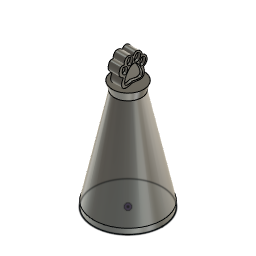
Pawn v1 (Autodesk Fusion 360 design; units mm, degrees)
Autodesk Fusion 360 part; units mm, degrees
sketch "Sketch1" plane through (0, 0, 0) normal (0, 0, 1) x (1, 0, 0)
  circle A0 centre (0, 0) radius 12.5
  dimension "d1" = 25
  constraint coincident A0.centre origin
  measures "d1" diameter of A0
extrude "Extrude2" add sketch "Sketch1" along normal blind 2 makes body 1
ref_plane "WorkPlane3" through (0, 0, 22) normal (0, 0, 1) x (1, 0, 0)
sketch "Sketch5" plane through (0, 0, 22) normal (0, 0, 1) x (1, 0, 0)
ref_plane "WorkPlane4" through (0, 0, 37) normal (0, 0, 1) x (1, 0, 0)
sketch "Sketch6" plane through (0, 0, 37) normal (0, 0, 1) x (1, 0, 0)
  circle A0 centre (0, 0) radius 5
  dimension "d11" = 10
  constraint coincident A0.centre origin
  measures "d11" diameter of A0
loft "Loft2" add profiles "Sketch6" section 1 section 2 face at (-3.3879, -0.621, 2) on bodies 1 bodies 1
sphere "SpherePrimitive1" add diameter 16 placed x (1, 0, 0) y (0, 0, -1) z (0, 1, 0) at (-0.1087, 0, 43.069) separate body makes body 2
move_body "Move1" bodies 2 to x (1, 0, 0) y (0, 1, 0) z (0, 0, 1) at (0, 0, 2)
ref_plane "WorkPlane5" through (0, 0, 40) normal (0, 0, 1) x (1, 0, 0)
ref_plane "WorkPlane6" through (0, 0, 40) normal (0, 0, 1) x (1, 0, 0)
sketch "Sketch9" plane through (0, 0, 40) normal (0, 0, 1) x (1, 0, 0)
  circle A0 centre (0, 0) radius 5.75
  dimension "d15" = 11.5
  constraint coincident A0.centre origin
  measures "d15" diameter of A0
loft "Loft3" add profiles "Sketch9" section 1 section 2 face at (1.3101, -1.9935, 37) on bodies 1 bodies 1
sketch "Sketch10" plane through (0, 0, 0) normal (1, 0, 0) x (0, 1, 0)
sketch "Sketch11" plane through (0, 0, 0) normal (1, 0, 0) x (0, 1, 0)
  spline S0 degree 5 poles (-3.2787, 40.0454) (-3.329, 40.0614) (-3.4264, 40.0962) (-3.5629, 40.1571) (-3.7251, 40.2561) (-3.8983, 40.4129) (-4.046, 40.6065) (-4.1701, 40.8394) (-4.2671, 41.1119) (-4.3286, 41.421) (-4.346, 41.7602) (-4.3129, 42.1194) (-4.2293, 42.4841) (-4.1045, 42.8352) (-3.9605, 43.1487) (-3.8264, 43.402) (-3.7324, 43.5808) (-3.7041, 43.6847) (-3.7567, 43.7354) (-3.8898, 43.7779) (-4.0914, 43.8587) (-4.3385, 44.0022) (-4.6016, 44.2078) (-4.8494, 44.461) (-5.0537, 44.7411) (-5.1943, 45.0301) (-5.2638, 45.3212) (-5.2715, 45.6253) (-5.2323, 45.9576) (-5.1613, 46.3292) (-5.0588, 46.7299) (-4.9167, 47.132) (-4.6743, 47.4432) (-4.3169, 47.6052) (-3.9101, 47.6407) (-3.5409, 47.6019) (-3.2925, 47.5555) (-3.2103, 47.5569) (-3.2577, 47.6187) (-3.3419, 47.7258) (-3.4015, 47.8936) (-3.4041, 48.1515) (-3.3297, 48.5128) (-3.1643, 48.9586) (-2.8776, 49.3926) (-2.4359, 49.6631) (-1.8831, 49.7359) (-1.2904, 49.6236) (-0.7461, 49.3872) (-0.3293, 49.108) (-0.0883, 48.8721) (-0.0225, 48.7508) (-0.0481, 48.7788) (-0.0376, 48.9475) (0.0779, 49.2091) (0.3231, 49.4918) (0.6879, 49.7166) (1.1382, 49.8139) (1.6263, 49.7381) (2.102, 49.4885) (2.5203, 49.1092) (2.8455, 48.6689) (3.056, 48.2458) (3.1485, 47.9102) (3.1443, 47.7074) (3.0901, 47.6442) (3.0717, 47.6629) (3.173, 47.6744) (3.413, 47.6175) (3.7661, 47.4522) (4.1752, 47.1612) (4.568, 46.7471) (4.8713, 46.2325) (5.0266, 45.6568) (5.0053, 45.0802) (4.8255, 44.5564) (4.5349, 44.1273) (4.1987, 43.8196) (3.8857, 43.6405) (3.6544, 43.573) (3.5411, 43.5739) (3.5419, 43.5636) (3.6213, 43.453) (3.7415, 43.2023) (3.8648, 42.8146) (3.9562, 42.323) (3.9849, 41.78) (3.9268, 41.2459) (3.7666, 40.778) (3.4996, 40.4189) (3.1339, 40.1852) (2.6877, 40.0725) (2.1856, 40.0606) (1.6557, 40.1193) (1.1259, 40.2132) (0.6213, 40.3077) (0.1604, 40.3737) (-0.248, 40.3937) (-0.607, 40.3654) (-0.9274, 40.2973) (-1.2242, 40.2048) (-1.5129, 40.1065) (-1.806, 40.0204) (-2.1092, 39.96) (-2.4188, 39.9314) (-2.7258, 39.936) (-2.9602, 39.9652) (-3.1247, 40.0003) (-3.2284, 40.0294) (-3.2787, 40.0454) knots 0 0 0 0 0 0 0.00952381 0.01904762 0.02857143 0.03809524 0.04761905 0.05714286 0.06666667 0.07619048 0.08571429 0.0952381 0.1047619 0.11428571 0.12380952 0.13333333 0.14285714 0.15238095 0.16190476 0.17142857 0.18095238 0.19047619 0.2 0.20952381 0.21904762 0.22857143 0.23809524 0.24761905 0.25714286 0.26666667 0.27619048 0.28571429 0.2952381 0.3047619 0.31428571 0.32380952 0.33333333 0.34285714 0.35238095 0.36190476 0.37142857 0.38095238 0.39047619 0.4 0.40952381 0.41904762 0.42857143 0.43809524 0.44761905 0.45714286 0.46666667 0.47619048 0.48571429 0.4952381 0.5047619 0.51428571 0.52380952 0.53333333 0.54285714 0.55238095 0.56190476 0.57142857 0.58095238 0.59047619 0.6 0.60952381 0.61904762 0.62857143 0.63809524 0.64761905 0.65714286 0.66666667 0.67619048 0.68571429 0.6952381 0.7047619 0.71428571 0.72380952 0.73333333 0.74285714 0.75238095 0.76190476 0.77142857 0.78095238 0.79047619 0.8 0.80952381 0.81904762 0.82857143 0.83809524 0.84761905 0.85714286 0.86666667 0.87619048 0.88571429 0.8952381 0.9047619 0.91428571 0.92380952 0.93333333 0.94285714 0.95238095 0.96190476 0.97142857 0.98095238 0.99047619 1 1 1 1 1 1
  line L0 (-4.3951, 46.9042) -> (-1.7589, 51.2055)
  line L1 (-6.0697, 44.8771) -> (-3.7447, 49.286)
  line L2 (4.2895, 48.7822) -> (5.6048, 42.9491)
  point P0 (-4.0893, 40.6991)
  point P1 (-4.2201, 42.4774)
  point P2 (-3.7232, 43.6541)
  point P3 (-3.9799, 43.8169)
  point P4 (-5.1582, 44.9824)
  point P5 (-4.9072, 47.0816)
  point P6 (-3.2787, 47.5628)
  point P7 (-3.2787, 47.6466)
  point P8 (-3.077, 49.0548)
  point P9 (-0.0768, 48.8344)
  point P10 (-0.0396, 48.8147)
  point P11 (1.3943, 49.7526)
  point P12 (3.1219, 47.7028)
  point P13 (3.0986, 47.6608)
  point P14 (4.9471, 45.8656)
  point P15 (3.6234, 43.5786)
  point P16 (3.5674, 43.5289)
  point P17 (3.7321, 40.79)
  point P18 (0.2661, 40.3525)
  point P19 (-1.7349, 40.0454)
  constraint midpoint P8 L0
  constraint midpoint P5 L1
  constraint midpoint P14 L2
extrude "Extrude3" add sketch "Sketch11" along normal mid plane 4 separate body contours S0 makes body 3
sketch "Sketch12" plane through (2, 0, 0) normal (1, 0, 0) x (0, 1, 0)
  spline S0 degree 5 poles (-3.2787, 40.0454) (-3.2284, 40.0294) (-3.1247, 40.0003) (-2.9602, 39.9652) (-2.7258, 39.936) (-2.4188, 39.9314) (-2.1092, 39.96) (-1.806, 40.0204) (-1.5129, 40.1065) (-1.2242, 40.2048) (-0.9274, 40.2973) (-0.607, 40.3654) (-0.248, 40.3937) (0.1604, 40.3737) (0.6213, 40.3077) (1.1259, 40.2132) (1.6557, 40.1193) (2.1856, 40.0606) (2.6877, 40.0725) (3.1339, 40.1852) (3.4996, 40.4189) (3.7666, 40.778) (3.9268, 41.2459) (3.9849, 41.78) (3.9562, 42.323) (3.8648, 42.8146) (3.7415, 43.2023) (3.6213, 43.453) (3.5419, 43.5636) (3.5411, 43.5739) (3.6544, 43.573) (3.8857, 43.6405) (4.1987, 43.8196) (4.5349, 44.1273) (4.8255, 44.5564) (5.0053, 45.0802) (5.0266, 45.6568) (4.8713, 46.2325) (4.568, 46.7471) (4.1752, 47.1612) (3.7661, 47.4522) (3.413, 47.6175) (3.207, 47.6664) (3.1242, 47.6667) (3.0991, 47.6613) (3.0931, 47.6593) (3.0922, 47.6589) knots -1 -1 -1 -1 -1 -1 -0.990476 -0.980952 -0.971429 -0.961905 -0.952381 -0.942857 -0.933333 -0.92381 -0.914286 -0.904762 -0.895238 -0.885714 -0.87619 -0.866667 -0.857143 -0.847619 -0.838095 -0.828571 -0.819048 -0.809524 -0.8 -0.790476 -0.780952 -0.771429 -0.761905 -0.752381 -0.742857 -0.733333 -0.72381 -0.714286 -0.704762 -0.695238 -0.685714 -0.67619 -0.666667 -0.657143 -0.647619 -0.638095 -0.628571 -0.619048 -0.609524 -0.606751 -0.606751 -0.606751 -0.606751 -0.606751 -0.606751
  spline S1 degree 5 poles (3.0922, 47.6589) (3.0916, 47.6586) (3.0911, 47.6584) (3.0908, 47.6582) (3.0906, 47.6582) (3.0906, 47.6582) knots 0.602912 0.602912 0.602912 0.602912 0.602912 0.602912 0.604832 0.604832 0.604832 0.604832 0.604832 0.604832
  spline S2 degree 5 poles (3.0922, 47.6589) (3.093, 47.6595) (3.098, 47.6627) (3.1148, 47.6778) (3.1449, 47.7356) (3.1485, 47.9102) (3.056, 48.2458) (2.8455, 48.6689) (2.5203, 49.1092) (2.102, 49.4885) (1.6263, 49.7381) (1.1382, 49.8139) (0.6879, 49.7166) (0.3231, 49.4918) (0.0779, 49.2091) (-0.0376, 48.9475) (-0.0481, 48.7788) (-0.0225, 48.7508) (-0.0883, 48.8721) (-0.3293, 49.108) (-0.7461, 49.3872) (-1.2904, 49.6236) (-1.8831, 49.7359) (-2.4359, 49.6631) (-2.8776, 49.3926) (-3.1643, 48.9586) (-3.3297, 48.5128) (-3.4041, 48.1515) (-3.4015, 47.8936) (-3.3419, 47.7258) (-3.2577, 47.6187) (-3.2103, 47.5569) (-3.2925, 47.5555) (-3.5409, 47.6019) (-3.9101, 47.6407) (-4.3169, 47.6052) (-4.6743, 47.4432) (-4.9167, 47.132) (-5.0588, 46.7299) (-5.1613, 46.3292) (-5.2323, 45.9576) (-5.2715, 45.6253) (-5.2638, 45.3212) (-5.1943, 45.0301) (-5.0537, 44.7411) (-4.8494, 44.461) (-4.6016, 44.2078) (-4.3385, 44.0022) (-4.0914, 43.8587) (-3.8898, 43.7779) (-3.7567, 43.7354) (-3.7041, 43.6847) (-3.7324, 43.5808) (-3.8264, 43.402) (-3.9605, 43.1487) (-4.1045, 42.8352) (-4.2293, 42.4841) (-4.3129, 42.1194) (-4.346, 41.7602) (-4.3286, 41.421) (-4.2671, 41.1119) (-4.1701, 40.8394) (-4.046, 40.6065) (-3.8983, 40.4129) (-3.7251, 40.2561) (-3.5629, 40.1571) (-3.4264, 40.0962) (-3.329, 40.0614) (-3.2787, 40.0454) knots -0.6029125 -0.6029125 -0.6029125 -0.6029125 -0.6029125 -0.6029125 -0.6 -0.59047619 -0.58095238 -0.57142857 -0.56190476 -0.55238095 -0.54285714 -0.53333333 -0.52380952 -0.51428571 -0.5047619 -0.4952381 -0.48571429 -0.47619048 -0.46666667 -0.45714286 -0.44761905 -0.43809524 -0.42857143 -0.41904762 -0.40952381 -0.4 -0.39047619 -0.38095238 -0.37142857 -0.36190476 -0.35238095 -0.34285714 -0.33333333 -0.32380952 -0.31428571 -0.3047619 -0.2952381 -0.28571429 -0.27619048 -0.26666667 -0.25714286 -0.24761905 -0.23809524 -0.22857143 -0.21904762 -0.20952381 -0.2 -0.19047619 -0.18095238 -0.17142857 -0.16190476 -0.15238095 -0.14285714 -0.13333333 -0.12380952 -0.11428571 -0.1047619 -0.0952381 -0.08571429 -0.07619048 -0.06666667 -0.05714286 -0.04761905 -0.03809524 -0.02857143 -0.01904762 -0.00952381 0 0 0 0 0 0
  spline S3 degree 5 poles (-3.2297, 41.5048) (-3.2452, 41.6006) (-3.2623, 41.8061) (-3.2457, 42.155) (-3.1382, 42.691) (-2.8727, 43.4345) (-2.4965, 44.1953) (-2.0362, 44.9126) (-1.5214, 45.5276) (-0.9815, 45.9909) (-0.4424, 46.2689) (0.077, 46.3523) (0.5652, 46.2543) (1.0161, 46.0028) (1.4279, 45.6334) (1.8016, 45.1835) (2.1396, 44.6841) (2.4446, 44.1565) (2.7175, 43.6152) (2.9562, 43.0715) (3.1541, 42.5358) (3.2984, 42.0212) (3.3682, 41.5458) (3.334, 41.1358) (3.1675, 40.818) (2.8534, 40.6125) (2.3983, 40.5259) (1.8441, 40.5432) (1.2558, 40.6325) (0.7041, 40.7544) (0.2482, 40.8694) (-0.0789, 40.9452) (-0.2918, 40.9665) (-0.4526, 40.9375) (-0.6349, 40.8731) (-0.8899, 40.7913) (-1.2271, 40.709) (-1.6295, 40.6444) (-2.0617, 40.6189) (-2.4809, 40.6591) (-2.8451, 40.797) (-3.0621, 41.0082) (-3.1695, 41.2314) (-3.2142, 41.409) (-3.2297, 41.5048) knots 0 0 0 0 0 0 0.025 0.05 0.075 0.1 0.125 0.15 0.175 0.2 0.225 0.25 0.275 0.3 0.325 0.35 0.375 0.4 0.425 0.45 0.475 0.5 0.525 0.55 0.575 0.6 0.625 0.65 0.675 0.7 0.725 0.75 0.775 0.8 0.825 0.85 0.875 0.9 0.925 0.95 0.975 1 1 1 1 1 1
  spline S4 degree 5 poles (-3.7437, 46.842) (-3.718, 46.8616) (-3.6659, 46.8927) (-3.5864, 46.9161) (-3.4795, 46.91) (-3.3455, 46.8724) (-3.2102, 46.8341) (-3.0717, 46.8093) (-2.9283, 46.787) (-2.7794, 46.7437) (-2.627, 46.6532) (-2.4764, 46.497) (-2.3377, 46.2748) (-2.2233, 45.9989) (-2.1461, 45.69) (-2.1179, 45.373) (-2.147, 45.0729) (-2.236, 44.8093) (-2.3814, 44.5951) (-2.5749, 44.4385) (-2.8042, 44.3439) (-3.0544, 44.3137) (-3.3091, 44.3499) (-3.551, 44.4549) (-3.764, 44.629) (-3.9342, 44.8691) (-4.0514, 45.1667) (-4.1104, 45.506) (-4.1132, 45.8617) (-4.067, 46.2029) (-3.9823, 46.4988) (-3.8935, 46.6788) (-3.8201, 46.7752) (-3.7694, 46.8225) (-3.7437, 46.842) knots 0 0 0 0 0 0 0.033333 0.066667 0.1 0.133333 0.166667 0.2 0.233333 0.266667 0.3 0.333333 0.366667 0.4 0.433333 0.466667 0.5 0.533333 0.566667 0.6 0.633333 0.666667 0.7 0.733333 0.766667 0.8 0.833333 0.866667 0.9 0.933333 0.966667 1 1 1 1 1 1
  spline S5 degree 5 poles (-1.6285, 48.9967) (-1.5819, 49.0042) (-1.484, 49.0136) (-1.3243, 49.0106) (-1.0928, 48.9719) (-0.7997, 48.8653) (-0.5341, 48.7022) (-0.3245, 48.4873) (-0.1913, 48.2283) (-0.139, 47.938) (-0.158, 47.6326) (-0.2306, 47.3298) (-0.3365, 47.047) (-0.4579, 46.7993) (-0.5853, 46.5976) (-0.7218, 46.4468) (-0.8763, 46.348) (-1.0578, 46.3002) (-1.2699, 46.3017) (-1.5037, 46.3525) (-1.7406, 46.453) (-1.9583, 46.6032) (-2.1359, 46.8011) (-2.2591, 47.0414) (-2.326, 47.3139) (-2.3434, 47.605) (-2.323, 47.8994) (-2.2764, 48.1814) (-2.2111, 48.4366) (-2.1255, 48.6536) (-2.0091, 48.8248) (-1.882, 48.9209) (-1.7638, 48.9686) (-1.6752, 48.9892) (-1.6285, 48.9967) knots 0 0 0 0 0 0 0.033333 0.066667 0.1 0.133333 0.166667 0.2 0.233333 0.266667 0.3 0.333333 0.366667 0.4 0.433333 0.466667 0.5 0.533333 0.566667 0.6 0.633333 0.666667 0.7 0.733333 0.766667 0.8 0.833333 0.866667 0.9 0.933333 0.966667 1 1 1 1 1 1
  spline S6 degree 5 poles (1.554, 48.9967) (1.5157, 49.0039) (1.4395, 49.0119) (1.3271, 49.004) (1.1816, 48.9521) (1.007, 48.8205) (0.84, 48.6289) (0.6831, 48.387) (0.5439, 48.1068) (0.4346, 47.8012) (0.3687, 47.4845) (0.359, 47.1715) (0.4147, 46.8775) (0.5386, 46.618) (0.7246, 46.4083) (0.959, 46.2623) (1.2242, 46.1906) (1.5005, 46.1986) (1.7693, 46.2849) (2.016, 46.4394) (2.2294, 46.6452) (2.4019, 46.8826) (2.5284, 47.1323) (2.6065, 47.3786) (2.6351, 47.6135) (2.6152, 47.8366) (2.5493, 48.051) (2.4418, 48.26) (2.299, 48.4635) (2.1294, 48.6543) (1.9424, 48.8193) (1.7864, 48.9188) (1.6695, 48.9686) (1.5924, 48.9895) (1.554, 48.9967) knots 0 0 0 0 0 0 0.033333 0.066667 0.1 0.133333 0.166667 0.2 0.233333 0.266667 0.3 0.333333 0.366667 0.4 0.433333 0.466667 0.5 0.533333 0.566667 0.6 0.633333 0.666667 0.7 0.733333 0.766667 0.8 0.833333 0.866667 0.9 0.933333 0.966667 1 1 1 1 1 1
  spline S7 degree 5 poles (3.4122, 46.842) (3.3551, 46.8469) (3.2415, 46.8457) (3.0754, 46.8119) (2.8703, 46.7064) (2.655, 46.4928) (2.4899, 46.2215) (2.3796, 45.9175) (2.3246, 45.6023) (2.3213, 45.2902) (2.3643, 44.991) (2.4472, 44.7125) (2.5644, 44.4624) (2.7127, 44.2509) (2.8922, 44.093) (3.1036, 44.0045) (3.3442, 43.9992) (3.6056, 44.0856) (3.8696, 44.2632) (4.1107, 44.5228) (4.3016, 44.8487) (4.4178, 45.2193) (4.4416, 45.6092) (4.368, 45.9898) (4.2064, 46.3314) (3.976, 46.606) (3.7566, 46.7536) (3.5843, 46.8168) (3.4693, 46.8372) (3.4122, 46.842) knots 0 0 0 0 0 0 0.04 0.08 0.12 0.16 0.2 0.24 0.28 0.32 0.36 0.4 0.44 0.48 0.52 0.56 0.6 0.64 0.68 0.72 0.76 0.8 0.84 0.88 0.92 0.96 1 1 1 1 1 1
  point P0 (-0.7785, 46.0711)
  point P1 (1.6924, 45.3002)
  point P2 (3.2738, 42.0583)
  point P3 (2.7401, 40.6153)
  point P4 (0.0517, 40.9118)
  point P5 (-0.5809, 40.892)
  point P6 (-1.9448, 40.6351)
  point P7 (-3.2297, 46.842)
  point P8 (-2.6367, 46.6444)
  point P9 (-2.1425, 45.2013)
  point P10 (-2.9925, 44.3316)
  point P11 (-4.0533, 45.2409)
  point P12 (-0.2843, 48.3839)
  point P13 (-0.4425, 46.842)
  point P14 (-1.1146, 46.3083)
  point P15 (-2.1425, 46.842)
  point P16 (-2.2413, 48.3048)
  point P17 (0.7633, 48.5025)
  point P18 (0.4471, 46.842)
  point P19 (1.554, 46.2293)
  point P20 (2.5622, 47.2572)
  point P21 (2.404, 48.3048)
  point P22 (2.404, 45.9525)
  point P23 (2.5622, 44.4897)
  point P24 (3.4122, 44.0351)
  point P25 (4.4203, 45.4781)
extrude "Extrude4" cut sketch "Sketch12" against normal blind 1 contours S3 | S4 | S5 | S6 | S7 bodies 3
sketch "Sketch13" plane through (-2, 0, 0) normal (-1, 0, 0) x (0, -1, 0)
  spline S0 degree 5 poles (-3.0922, 47.6589) (-3.0931, 47.6593) (-3.0991, 47.6613) (-3.1242, 47.6667) (-3.207, 47.6664) (-3.413, 47.6175) (-3.7661, 47.4522) (-4.1752, 47.1612) (-4.568, 46.7471) (-4.8713, 46.2325) (-5.0266, 45.6568) (-5.0053, 45.0802) (-4.8255, 44.5564) (-4.5349, 44.1273) (-4.1987, 43.8196) (-3.8857, 43.6405) (-3.6544, 43.573) (-3.5411, 43.5739) (-3.5419, 43.5636) (-3.6213, 43.453) (-3.7415, 43.2023) (-3.8648, 42.8146) (-3.9562, 42.323) (-3.9849, 41.78) (-3.9268, 41.2459) (-3.7666, 40.778) (-3.4996, 40.4189) (-3.1339, 40.1852) (-2.6877, 40.0725) (-2.1856, 40.0606) (-1.6557, 40.1193) (-1.1259, 40.2132) (-0.6213, 40.3077) (-0.1604, 40.3737) (0.248, 40.3937) (0.607, 40.3654) (0.9274, 40.2973) (1.2242, 40.2048) (1.5129, 40.1065) (1.806, 40.0204) (2.1092, 39.96) (2.4188, 39.9314) (2.7258, 39.936) (2.9602, 39.9652) (3.1247, 40.0003) (3.2284, 40.0294) (3.2787, 40.0454) knots 0.606751 0.606751 0.606751 0.606751 0.606751 0.606751 0.609524 0.619048 0.628571 0.638095 0.647619 0.657143 0.666667 0.67619 0.685714 0.695238 0.704762 0.714286 0.72381 0.733333 0.742857 0.752381 0.761905 0.771429 0.780952 0.790476 0.8 0.809524 0.819048 0.828571 0.838095 0.847619 0.857143 0.866667 0.87619 0.885714 0.895238 0.904762 0.914286 0.92381 0.933333 0.942857 0.952381 0.961905 0.971429 0.980952 0.990476 1 1 1 1 1 1
  spline S1 degree 5 poles (3.2787, 40.0454) (3.329, 40.0614) (3.4264, 40.0962) (3.5629, 40.1571) (3.7251, 40.2561) (3.8983, 40.4129) (4.046, 40.6065) (4.1701, 40.8394) (4.2671, 41.1119) (4.3286, 41.421) (4.346, 41.7602) (4.3129, 42.1194) (4.2293, 42.4841) (4.1045, 42.8352) (3.9605, 43.1487) (3.8264, 43.402) (3.7324, 43.5808) (3.7041, 43.6847) (3.7567, 43.7354) (3.8898, 43.7779) (4.0914, 43.8587) (4.3385, 44.0022) (4.6016, 44.2078) (4.8494, 44.461) (5.0537, 44.7411) (5.1943, 45.0301) (5.2638, 45.3212) (5.2715, 45.6253) (5.2323, 45.9576) (5.1613, 46.3292) (5.0588, 46.7299) (4.9167, 47.132) (4.6743, 47.4432) (4.3169, 47.6052) (3.9101, 47.6407) (3.5409, 47.6019) (3.2925, 47.5555) (3.2103, 47.5569) (3.2577, 47.6187) (3.3419, 47.7258) (3.4015, 47.8936) (3.4041, 48.1515) (3.3297, 48.5128) (3.1643, 48.9586) (2.8776, 49.3926) (2.4359, 49.6631) (1.8831, 49.7359) (1.2904, 49.6236) (0.7461, 49.3872) (0.3293, 49.108) (0.0883, 48.8721) (0.0225, 48.7508) (0.0481, 48.7788) (0.0376, 48.9475) (-0.0779, 49.2091) (-0.3231, 49.4918) (-0.6879, 49.7166) (-1.1382, 49.8139) (-1.6263, 49.7381) (-2.102, 49.4885) (-2.5203, 49.1092) (-2.8455, 48.6689) (-3.056, 48.2458) (-3.1485, 47.9102) (-3.1449, 47.7356) (-3.1148, 47.6778) (-3.098, 47.6627) (-3.093, 47.6595) (-3.0922, 47.6589) knots 0 0 0 0 0 0 0.00952381 0.01904762 0.02857143 0.03809524 0.04761905 0.05714286 0.06666667 0.07619048 0.08571429 0.0952381 0.1047619 0.11428571 0.12380952 0.13333333 0.14285714 0.15238095 0.16190476 0.17142857 0.18095238 0.19047619 0.2 0.20952381 0.21904762 0.22857143 0.23809524 0.24761905 0.25714286 0.26666667 0.27619048 0.28571429 0.2952381 0.3047619 0.31428571 0.32380952 0.33333333 0.34285714 0.35238095 0.36190476 0.37142857 0.38095238 0.39047619 0.4 0.40952381 0.41904762 0.42857143 0.43809524 0.44761905 0.45714286 0.46666667 0.47619048 0.48571429 0.4952381 0.5047619 0.51428571 0.52380952 0.53333333 0.54285714 0.55238095 0.56190476 0.57142857 0.58095238 0.59047619 0.6 0.6029125 0.6029125 0.6029125 0.6029125 0.6029125 0.6029125
  spline S2 degree 5 poles (-3.0922, 47.6589) (-3.0915, 47.6587) (-3.091, 47.6585) (-3.0907, 47.6583) (-3.0906, 47.6582) (-3.0906, 47.6582) knots -0.606751 -0.606751 -0.606751 -0.606751 -0.606751 -0.606751 -0.604832 -0.604832 -0.604832 -0.604832 -0.604832 -0.604832
  spline S3 degree 5 poles (-3.3971, 46.9773) (-3.4474, 46.9825) (-3.5491, 46.9821) (-3.7037, 46.9483) (-3.9065, 46.8346) (-4.1331, 46.585) (-4.3105, 46.2449) (-4.4194, 45.8398) (-4.4468, 45.4019) (-4.3899, 44.9689) (-4.254, 44.5795) (-4.0514, 44.2696) (-3.799, 44.0669) (-3.5168, 43.9874) (-3.2266, 44.0294) (-2.9496, 44.1728) (-2.7056, 44.3881) (-2.5107, 44.6431) (-2.3761, 44.9102) (-2.306, 45.1747) (-2.2973, 45.4361) (-2.3432, 45.6998) (-2.4351, 45.971) (-2.5651, 46.2485) (-2.7289, 46.5171) (-2.924, 46.7517) (-3.1028, 46.8889) (-3.2473, 46.9512) (-3.3468, 46.9722) (-3.3971, 46.9773) knots 0 0 0 0 0 0 0.04 0.08 0.12 0.16 0.2 0.24 0.28 0.32 0.36 0.4 0.44 0.48 0.52 0.56 0.6 0.64 0.68 0.72 0.76 0.8 0.84 0.88 0.92 0.96 1 1 1 1 1 1
  spline S4 degree 5 poles (-1.618, 48.9541) (-1.68, 48.9593) (-1.8013, 48.9512) (-1.972, 48.8839) (-2.1682, 48.6907) (-2.3479, 48.3211) (-2.4551, 47.8809) (-2.4871, 47.4301) (-2.4433, 47.0189) (-2.323, 46.6761) (-2.128, 46.415) (-1.8655, 46.24) (-1.5509, 46.1519) (-1.2113, 46.1545) (-0.8868, 46.258) (-0.621, 46.4711) (-0.4531, 46.7944) (-0.4101, 47.2141) (-0.4964, 47.6926) (-0.6948, 48.1722) (-0.9748, 48.5884) (-1.2334, 48.8218) (-1.4292, 48.9201) (-1.556, 48.9489) (-1.618, 48.9541) knots 0 0 0 0 0 0 0.05 0.1 0.15 0.2 0.25 0.3 0.35 0.4 0.45 0.5 0.55 0.6 0.65 0.7 0.75 0.8 0.85 0.9 0.95 1 1 1 1 1 1
  spline S5 degree 5 poles (1.5843, 48.9541) (1.5368, 48.966) (1.4386, 48.9837) (1.2832, 48.991) (1.0657, 48.9604) (0.7954, 48.8546) (0.5473, 48.6846) (0.3408, 48.4579) (0.1922, 48.1857) (0.1115, 47.8837) (0.1023, 47.5703) (0.1627, 47.265) (0.2862, 46.9864) (0.4625, 46.7503) (0.6779, 46.5677) (0.9164, 46.443) (1.1613, 46.376) (1.3969, 46.363) (1.6104, 46.3985) (1.7938, 46.4766) (1.945, 46.5923) (2.0662, 46.7412) (2.1612, 46.9191) (2.2338, 47.122) (2.2853, 47.3452) (2.3145, 47.5834) (2.3186, 47.8306) (2.2934, 48.0792) (2.2344, 48.3199) (2.1369, 48.5415) (1.9974, 48.7316) (1.8514, 48.8487) (1.7238, 48.912) (1.6319, 48.9421) (1.5843, 48.9541) knots 0 0 0 0 0 0 0.033333 0.066667 0.1 0.133333 0.166667 0.2 0.233333 0.266667 0.3 0.333333 0.366667 0.4 0.433333 0.466667 0.5 0.533333 0.566667 0.6 0.633333 0.666667 0.7 0.733333 0.766667 0.8 0.833333 0.866667 0.9 0.933333 0.966667 1 1 1 1 1 1
  spline S6 degree 5 poles (3.6401, 46.7994) (3.6041, 46.8347) (3.5299, 46.8977) (3.4131, 46.968) (3.2492, 47.0107) (3.0371, 46.9776) (2.8247, 46.8621) (2.6204, 46.6725) (2.4362, 46.4213) (2.2866, 46.1238) (2.1859, 45.7976) (2.1465, 45.4618) (2.1762, 45.1358) (2.2761, 44.839) (2.4395, 44.5896) (2.6537, 44.4035) (2.902, 44.2935) (3.1655, 44.2679) (3.4245, 44.3294) (3.6603, 44.4744) (3.8562, 44.6941) (3.9988, 44.975) (4.0796, 45.2999) (4.0959, 45.648) (4.0517, 45.9965) (3.9549, 46.322) (3.8436, 46.5463) (3.7461, 46.6858) (3.6762, 46.7641) (3.6401, 46.7994) knots 0 0 0 0 0 0 0.04 0.08 0.12 0.16 0.2 0.24 0.28 0.32 0.36 0.4 0.44 0.48 0.52 0.56 0.6 0.64 0.68 0.72 0.76 0.8 0.84 0.88 0.92 0.96 1 1 1 1 1 1
  spline S7 degree 5 poles (0.0029, 46.2657) (-0.0696, 46.267) (-0.2133, 46.2596) (-0.4247, 46.2201) (-0.6981, 46.1193) (-1.0253, 45.9334) (-1.3386, 45.7028) (-1.6407, 45.4344) (-1.937, 45.1218) (-2.2331, 44.7522) (-2.5307, 44.313) (-2.8244, 43.799) (-3.0985, 43.2186) (-3.3223, 42.6029) (-3.4564, 41.9986) (-3.4628, 41.4575) (-3.3137, 41.0267) (-3.0001, 40.7395) (-2.5427, 40.6034) (-1.9929, 40.5975) (-1.4143, 40.683) (-0.8684, 40.8121) (-0.4, 40.9362) (-0.0202, 41.0157) (0.3039, 41.0271) (0.6232, 40.9643) (0.9864, 40.8393) (1.4154, 40.6844) (1.8871, 40.5516) (2.3524, 40.5) (2.7521, 40.5838) (3.0318, 40.8402) (3.1616, 41.2754) (3.1385, 41.8647) (2.9773, 42.5633) (2.7057, 43.314) (2.3572, 44.0565) (1.9656, 44.7349) (1.5579, 45.3075) (1.1506, 45.7518) (0.753, 46.0598) (0.4459, 46.2002) (0.222, 46.2516) (0.0755, 46.2644) (0.0029, 46.2657) knots 0 0 0 0 0 0 0.025 0.05 0.075 0.1 0.125 0.15 0.175 0.2 0.225 0.25 0.275 0.3 0.325 0.35 0.375 0.4 0.425 0.45 0.475 0.5 0.525 0.55 0.575 0.6 0.625 0.65 0.675 0.7 0.725 0.75 0.775 0.8 0.825 0.85 0.875 0.9 0.925 0.95 0.975 1 1 1 1 1 1
  point P0 (-4.4052, 45.7913)
  point P1 (-3.6145, 44.032)
  point P2 (-2.4483, 44.7831)
  point P3 (-2.468, 46.0285)
  point P4 (-2.468, 47.432)
  point P5 (-1.618, 46.1866)
  point P6 (-0.4517, 46.9773)
  point P7 (0.2994, 48.3611)
  point P8 (0.4576, 46.7797)
  point P9 (1.5843, 46.4041)
  point P10 (2.1773, 46.9773)
  point P11 (2.2762, 48.1238)
  point P12 (2.7704, 46.7994)
  point P13 (2.1773, 45.2378)
  point P14 (3.0669, 44.2889)
  point P15 (4.0355, 45.1587)
  point P16 (-1.361, 45.6727)
  point P17 (-2.8831, 43.6564)
  point P18 (-3.1006, 40.8692)
  point P19 (-0.4913, 40.9087)
  point P20 (0.9518, 40.8494)
  point P21 (2.8494, 40.711)
  point P22 (2.0983, 44.4866)
extrude "Extrude5" cut sketch "Sketch13" against normal blind 1 contours S3 | S4 | S5 | S6 | S7 bodies 3
sketch "Sketch14" plane through (0, 0, 0) normal (0, 0, 1) x (1, 0, 0)
sketch "Sketch15" plane through (0, 0, 0) normal (0, 1, 0) x (1, 0, 0)
sketch "Sketch16" plane through (0, 0, 0) normal (1, 0, 0) x (0, 1, 0)
sketch "Sketch17" plane through (0, 0, 0) normal (0, 0, 1) x (1, 0, 0)
  line L0 (-9.6823, 12.7908) -> (8.4137, 12.7908) construction
  line L1 (8.4137, 12.7908) -> (8.4137, -3.5699) construction
  line L2 (8.4137, -3.5699) -> (-9.6823, -3.5699) construction
  line L3 (-9.6823, -3.5699) -> (-9.6823, 12.7908) construction
  dimension "d24" = 7
  text T0 "CAL" font "Arial" height 7 align left top in box 18.096 x 16.3608 at (-9.6823, 12.7908) x (1, 0) y (0, -1) spacing 1
extrude "Extrude6" cut sketch "Sketch17" along normal blind 3 text T0 bodies 1
hidden bodies 2
